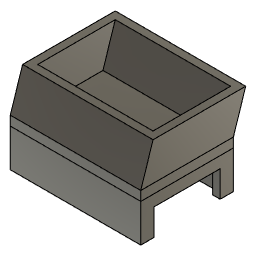
halterung für vorne v4 (Autodesk Fusion 360 design; units mm, degrees)
Autodesk Fusion 360 part; units mm, degrees
note: some values were not read from the file. Set by a fixed rule: which sketch regions a step uses.
sketch "Skizze18" plane through (0, 0, 0) normal (0, 0, 1) x (1, 0, 0)
  line L0 (34.5, 50.5) -> (-34.5, 50.5)
  line L1 (-34.5, 50.5) -> (-34.5, 99.5)
  line L2 (-34.5, 99.5) -> (34.5, 99.5)
  line L3 (34.5, 99.5) -> (34.5, 50.5)
  line L4 (34.5, 50.5) -> (-34.5, 99.5) construction
  line L5 (-34.5, 50.5) -> (34.5, 99.5) construction
  point P0 (0, 75)
  dimension "d92" = 69
  dimension "d93" = 49
  constraint perpendicular L0 L1
  constraint parallel L0 L2
  constraint parallel L1 L3
  constraint horizontal L0
  constraint coincident L4 P0
  constraint coincident L5 P0
  measures "d92" distance of L1.end L2.end
  measures "d93" distance of L0.end L1.end
extrude "Extrusion27" add sketch "Skizze18" along normal blind 20 makes body 1
sketch "Skizze19" plane through (0, 0, 20) normal (0, 0, 1) x (-1, 0, 0)
  line L0 (-34.5, -99.5) -> (34.5, -99.5)
  line L1 (34.5, -99.5) -> (34.5, -50.5)
  line L2 (34.5, -50.5) -> (-34.5, -50.5)
  line L3 (-34.5, -50.5) -> (-34.5, -99.5)
  line L4 (-30.5, -95.5) -> (30.5, -95.5)
  line L5 (30.5, -95.5) -> (30.5, -54.5)
  line L6 (30.5, -54.5) -> (-30.5, -54.5)
  line L7 (-30.5, -54.5) -> (-30.5, -95.5)
  line L8 (-30.5, -95.5) -> (30.5, -54.5) construction
  line L9 (30.5, -95.5) -> (-30.5, -54.5) construction
  point P0 (0, -75)
  dimension "d96" = 61
  dimension "d97" = 41
  constraint perpendicular L4 L5
  constraint parallel L4 L6
  constraint parallel L5 L7
  constraint horizontal L4
  constraint coincident L8 P0
  constraint coincident L9 P0
  measures "d96" distance of L5.end L6.end
  measures "d97" distance of L4.end L5.end
extrude "Extrusion28" cut sketch "Skizze19" against normal blind 20 contours L4 L5 L6 L7 bodies 1
extrude "Extrusion29" add 1 faces at (-10.1667, 98.1667, 20) along direction (0, 0, 1) blind 5 separate body on bodies 1 makes body 2
extrude "Extrusion30" add 1 faces at (30.5, 68.1667, 23.3333) along direction (-1, 0, 0) blind 61 separate body on bodies 2 makes body 3
extrude "Extrusion31" add 1 faces at (-10.1667, 98.1667, 25) along direction (0, 0, 1) blind 20 separate body on bodies 2 makes body 4
draft "Entwurf2" angle -18 neutral plane through (30.5, 54.5, 25) pull (0, 0, 1) 1 faces at (-11.5, 99.5, 31.6667) on bodies 4
draft "Entwurf3" angle -18 neutral plane through (30.5, 54.5, 25) pull (0, 0, 1) 1 faces at (-10.1667, 54.5, 31.6667) on bodies 4
draft "Entwurf4" angle 18 neutral plane through (30.5, 54.5, 25) pull (0, 0, 1) 1 faces at (11.5, 50.5, 31.6667) on bodies 4
draft "Entwurf5" angle 18 neutral plane through (30.5, 54.5, 25) pull (0, 0, 1) 1 faces at (10.1667, 95.5, 31.6667) on bodies 4
sketch "Skizze20" plane through (34.5, 0, 0) normal (1, 0, 0) x (0, 1, 0)
  line L0 (50.5, 0) -> (99.5, 0)
  line L1 (99.5, 0) -> (99.5, 20)
  line L2 (99.5, 20) -> (50.5, 20)
  line L3 (50.5, 20) -> (50.5, 0)
  circle A0 centre (75, 5) radius 5
  dimension "d116" = 10
  measures "d116" diameter of A0
extrude "Extrusion32" cut sketch "Skizze20" against normal blind 30 contours A0 bodies 1
sketch "Skizze21" plane through (34.5, 0, 0) normal (1, 0, 0) x (0, 1, 0)
  line L0 (75, 0) -> (99.5, 0)
  line L1 (99.5, 0) -> (99.5, 20)
  line L2 (99.5, 20) -> (50.5, 20)
  line L3 (50.5, 20) -> (50.5, 0)
  line L4 (50.5, 0) -> (75, 0)
  circle A0 centre (75, 5) radius 5
  line L5 (70.0006, 4.9232) -> (80, 4.9232)
  line L6 (80, 4.9232) -> (80, 0)
  line L7 (80, 0) -> (70.0006, 0)
  line L8 (70.0006, 0) -> (70.0006, 4.9232)
  constraint horizontal L5
  constraint vertical L6
  constraint horizontal L7
  constraint vertical L8
  constraint coincident L0 L6.end
  constraint coincident A0 L5.start
extrude "Extrusion33" cut sketch "Skizze21" against normal blind 30 contours L0 A0 L6 L7 | L4 A0 L7 L8 bodies 1
sketch "Skizze22" plane through (34.5, 0, 0) normal (1, 0, 0) x (0, 1, 0)
  line L0 (70.0006, 0) -> (70.0006, 4.9232)
  arc A0 (79.9994, 4.9232) -> (70.0006, 4.9232) centre (75, 5) ccw
  line L1 (79.9994, 4.9232) -> (80, 4.9232)
  line L2 (80, 4.9232) -> (80, 0)
  line L3 (80, 0) -> (99.5, 0)
  line L4 (99.5, 0) -> (99.5, 20)
  line L5 (99.5, 20) -> (50.5, 20)
  line L6 (50.5, 20) -> (50.5, 0)
  line L7 (50.5, 0) -> (70.0006, 0)
  line L8 (92.5, 10) -> (57.5, 10)
  line L9 (57.5, 10) -> (57.5, 0)
  line L10 (57.5, 0) -> (92.5, 0)
  line L11 (92.5, 0) -> (92.5, 10)
  line L12 (92.5, 10) -> (57.5, 0) construction
  line L13 (57.5, 10) -> (92.5, 0) construction
  line L14 (57.5, 10) -> (92.5, 10)
  line L15 (92.5, 10) -> (92.5, 14)
  line L16 (92.5, 14) -> (57.5, 14)
  line L17 (57.5, 14) -> (57.5, 10)
  point P0 (75, 5)
  dimension "d121" = 35
  dimension "d122" = 35
  constraint perpendicular L8 L9
  constraint parallel L8 L10
  constraint parallel L9 L11
  constraint horizontal L8
  constraint coincident L12 P0
  constraint coincident L13 P0
  constraint coincident P0 A0.centre
  constraint horizontal L14
  constraint vertical L15
  constraint horizontal L16
  constraint vertical L17
  measures "d121" distance of L9.end L10.end
  measures "d122" distance of L8.end L8.start
extrude "Extrusion34" cut sketch "Skizze22" against normal blind 7 contours L0 A0 L7 L8 L9 L10 L14 | A0 L2 L3 L8 L10 L11 L14 | L8 L14 L15 L16 L17 bodies 1
